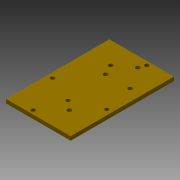
# Autodesk Inventor part: Z Rail
Saved by Autodesk Inventor 2013 SP2 (Build 170200200, 200)
## iProperties
Created: 2017-01-25
Part Number: Z Rail
Material: Generic
Document SubType Name: Modeling
Designer: Herman de Vries
Density: 1 g/cm^3
Mass: 14.7188 g
Surface Area: 110.688 cm^2
Volume: 14.7188 cm^3
Author: Herman de Vries
Autodesk Inventor part; units mm, degrees
ref_plane "YZ Plane" through (0, 0, 0) normal (1, 0, 0) x (0, 1, 0)
ref_plane "XZ Plane" through (0, 0, 0) normal (0, 1, 0) x (-1, 0, 0)
ref_plane "XY Plane" through (0, 0, 0) normal (0, 0, 1) x (1, 0, 0)
sketch "Sketch1" plane through (0, 0, 0) normal (0, 1, 0) x (-1, 0, 0)
  line L0 (0, 0) -> (50, 0)
  line L1 (50, 0) -> (50, 3)
  line L2 (50, 3) -> (0, 3)
  line L3 (0, 3) -> (0, 0)
  dimension "d0" = 50
  dimension "d1" = 3
  constraints: 8 end point, 2 parallel, 1 horizontal, 1 perpendicular
  measures "d0" distance of L2.end L1.end
  measures "d1" distance of L1.end L0.end
extrude "Extrusion1" add sketch "Sketch1" along normal blind 80
sketch "Sketch2" plane through (-50, 0, 3) normal (0, 0, 1) x (1, 0, 0)
  line L0 (0, 0) -> (0, 80) projected
  line L1 (50, 0) -> (50, 80) projected
  line L2 (0, 80) -> (50, 80) projected
  line L3 (50, 40) -> (40, 40)
  line L4 (40, 40) -> (40, 30)
  line L5 (40, 30) -> (50, 30)
  line L6 (50, 30) -> (50, 40)
  circle A0 centre (4, 32) radius 1.5 projected
  circle A1 centre (46, 32) radius 1.5 projected
  circle A2 centre (18, 63) radius 1.6 projected
  circle A3 centre (32, 77) radius 1.6 projected
  circle A4 centre (32, 17) radius 1.6 projected
  circle A5 centre (18, 3) radius 1.6 projected
  circle A6 centre (22, 55) radius 1.6 projected
  circle A7 centre (41, 55) radius 1.6 projected
  circle A8 centre (30, 72) radius 1.6 projected
  line L7 (0, 0) -> (50, 0) projected
  circle A9 centre (25, 23) radius 1.5
  point P0 (25, 80)
  point P1 (25, 0)
  dimension "d13" = 10
  dimension "d14" = 10
  dimension "d15" = 30
  dimension "d16" = 3
  dimension "d17" = 23
  constraints: 8 end point, 3 midpoint, 2 parallel, 1 centre point, 1 horizontal, 1 perpendicular, 1 vertical alignment
  measures "d13" distance of L3.start L3.end
  measures "d14" distance of L3.end L4.end
  measures "d15" distance from line of L1.start L5
  measures "d16" diameter of A9
  measures "d17" distance from line of L7 A9.centre
extrude "Extrusion2" cut sketch "Sketch2" against normal blind 5 contours A0 | A1 | A2 | A3 | A4 | A5 | A6 | A7 | A8 | A9
body "Solid1"
